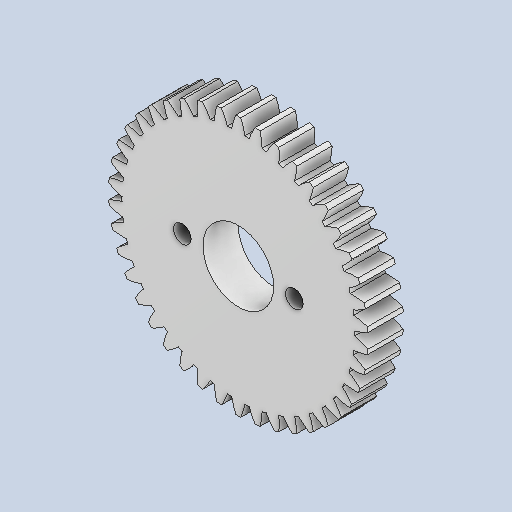
# Autodesk Inventor part: 平歯車2
Saved by Autodesk Inventor 2025.2 (Build 292293000, 293)
## iProperties
CustomPartVersion: 1
Created: 2025-01-07
Part Number: 平歯車2
Material: ABS プラスチック
Document SubType Name: Modeling
Designer: haruy
Categories: <?xml version="1.0" encoding="UTF-16"?> <MemberInstance><Categories><FamilyTemplate><FamilyTemplateParameter ValueType="xs:double" Id="1" ObjectReferenceKey="da_z" ObjectType="kUserParameterObject"/><FamilyTemplateParameter ValueType="xs:double" Id="2" ObjectReferenceKey="da_b" ObjectType="kUserParameterObject"/><FamilyTemplateParameter ValueType="xs:double" Id="3" ObjectReferenceKey="da_beta" ObjectType="kUserParameterObject"/><FamilyTemplateParameter ValueType="xs:double" Id="4" ObjectReferenceKey="da_da" ObjectType="kUserParameterObject"/><FamilyTemplateParameter ValueType="xs:double" Id="5" ObjectReferenceKey="da_aw" ObjectType="kUserParameterObject"/><FamilyTemplateParameter ValueType="xs:string" Id="6" ObjectReferenceKey="EAIAABAAAACIAQAAAAAAAIAAAAAAAAAA" ObjectType="83910656" SubObjectId="SurfaceGeometry"/></FamilyTemplate><ParamToTemplateMap><ParamToTemplate CategoryParameter="//CategoryParameter[@InternalName='046C89C9-8512-4d59-83FE-43B91F4F132A']" TemplateParameter="1"/><ParamToTemplate CategoryParameter="//CategoryParameter[@InternalName='2552DF32-E462-4b46-AEBF-C6C7768E72AC']" TemplateParameter="2"/><ParamToTemplate CategoryParameter="//CategoryParameter[@InternalName='C9EE641D-15FC-4fae-A226-E94C4372FDD7']" TemplateParameter="3"/><ParamToTemplate><ParamToTemplate CategoryParameter="//CategoryParameter[@InternalName='00B6519A-459B-49c7-AD84-2E56D39A5744']" ConstantValue="0.000000"/></ParamToTemplate><ParamToTemplate><ParamToTemplate CategoryParameter="//CategoryParameter[@InternalName='04B31F0E-C7A6-4894-AA32-9629BEFACF47']" ConstantValue="1.000000"/></ParamToTemplate><ParamToTemplate><ParamToTemplate CategoryParameter="//CategoryParameter[@InternalName='43CBEC2E-7847-49e7-A936-2F7889FCB2D9']" ConstantValue="0.250000"/></ParamToTemplate><ParamToTemplate><ParamToTemplate CategoryParameter="//CategoryParameter[@InternalName='B1EFC894-105D-4ebd-86BF-FA20ED196853']" ConstantValue="0.350000"/></ParamToTemplate><ParamToTemplate><ParamToTemplate CategoryParameter="//CategoryParameter[@InternalName='51175063-3D10-4879-93E8-6246FE8B403D']" ConstantValue="2060000000.000000"/></ParamToTemplate><ParamToTemplate><ParamToTemplate CategoryParameter="//CategoryParameter[@InternalName='A3A52E27-4454-46a9-B0BD-C932399B70AF']" ConstantValue="0.300000"/></ParamToTemplate><ParamToTemplate><ParamToTemplate CategoryParameter="//CategoryParameter[@InternalName='91B76062-C214-41d9-B1B9-14D2AB99603D']" ConstantValue="0.100000"/></ParamToTemplate><ParamToTemplate><ParamToTemplate CategoryParameter="//CategoryParameter[@InternalName='374E806E-8B8A-4dda-A9AA-1039D6500AD2']" ConstantValue="10.000000"/></ParamToTemplate><ParamToTemplate><ParamToTemplate CategoryParameter="//CategoryParameter[@InternalName='2D373A89-B862-43d6-8D0B-0CBF12AB9F6C']" ConstantValue="0.349066"/></ParamToTemplate><ParamToTemplate CategoryParameter="//CategoryParameter[@InternalName='37777632-D6A2-4fac-9D53-DB8ACD95C989']" TemplateParameter="4"/><ParamToTemplate CategoryParameter="//CategoryParameter[@InternalName='FD1017F1-B727-4f7e-9707-0F86F1FF9423']" TemplateParameter="5"/><ParamToTemplate><ParamToTemplate CategoryParameter="//CategoryParameter[@InternalName='9E1B4470-B2D3-4ff1-B813-535BB4CDF51A']" ConstantValue="3520000.000000"/></ParamToTemplate><ParamToTemplate><ParamToTemplate CategoryParameter="//CategoryParameter[@InternalName='F8452263-BFF6-458c-9FB1-07C4B99E95CD']" ConstantValue="11400000.000000"/></ParamToTemplate><ParamToTemplate><ParamToTemplate CategoryParameter="//CategoryParameter[@InternalName='3E3BB259-FD49-497f-8171-6EBC954A3479']" ConstantValue="2.000000"/></ParamToTemplate><ParamToTemplate CategoryParameter="//CategoryParameter[@InternalName='27C3BAF2-7550-4e4b-AE2C-0DB134B7D9B7']" TemplateParameter="6"/></ParamToTemplateMap><Category DisplayName="Gear" InternalName="DC85795E-93AB-48d5-8EEE-5A27447B64BD" Mnemonic="Gear"><CategoryParameter DisplayName="z" InternalName="046C89C9-8512-4d59-83FE-43B91F4F132A" Mnemonic="z"/><CategoryParameter DisplayName="b" InternalName="2552DF32-E462-4b46-AEBF-C6C7768E72AC" Mnemonic="b"/><CategoryParameter DisplayName="||b|" InternalName="C9EE641D-15FC-4fae-A226-E94C4372FDD7" Mnemonic="beta"/><CategoryParameter DisplayName="x" InternalName="00B6519A-459B-49c7-AD84-2E56D39A5744" Mnemonic="x"/><CategoryParameter DisplayName="a*" InternalName="04B31F0E-C7A6-4894-AA32-9629BEFACF47" Mnemonic="a"/><CategoryParameter DisplayName="c*" InternalName="43CBEC2E-7847-49e7-A936-2F7889FCB2D9" Mnemonic="c"/><CategoryParameter DisplayName="r|.f|*" InternalName="B1EFC894-105D-4ebd-86BF-FA20ED196853" Mnemonic="rf"/><CategoryParameter DisplayName="E" InternalName="51175063-3D10-4879-93E8-6246FE8B403D" Mnemonic="E"/><CategoryParameter DisplayName="||m|" InternalName="A3A52E27-4454-46a9-B0BD-C932399B70AF" Mnemonic="mi"/><Category DisplayName="SpurGear" InternalName="26C5A22E-A91E-4dfd-A3B3-23CCAFAE1764" Mnemonic="SpurGear"><CategoryParameter DisplayName="m" InternalName="91B76062-C214-41d9-B1B9-14D2AB99603D" Mnemonic="m"/><CategoryParameter DisplayName="P" InternalName="374E806E-8B8A-4dda-A9AA-1039D6500AD2" Mnemonic="PP"/><CategoryParameter DisplayName="||a|" InternalName="2D373A89-B862-43d6-8D0B-0CBF12AB9F6C" Mnemonic="alpha"/><CategoryParameter DisplayName="d|.a|" InternalName="37777632-D6A2-4fac-9D53-DB8ACD95C989" Mnemonic="da"/><CategoryParameter DisplayName="a|.w|" InternalName="FD1017F1-B727-4f7e-9707-0F86F1FF9423" Mnemonic="aw"/><CategoryParameter DisplayName="||s||.Flim|" InternalName="9E1B4470-B2D3-4ff1-B813-535BB4CDF51A" Mnemonic="sFlim"/><CategoryParameter DisplayName="||s||.Hlim|" InternalName="F8452263-BFF6-458c-9FB1-07C4B99E95CD" Mnemonic="sHlim"/><CategoryParameter DisplayName="タイプ" InternalName="3E3BB259-FD49-497f-8171-6EBC954A3479" Mnemonic="type"/><CategoryParameter DisplayName="PitchDiameter" InternalName="27C3BAF2-7550-4e4b-AE2C-0DB134B7D9B7" Mnemonic="IDS_PITCHDIAM"/></Category></Category></Categories></MemberInstance>
Density: 1.06 g/cm^3
Appearance: 滑らか - 白
Mass: 64.8659 g
Surface Area: 43.5022 cm^2
Volume: 8.26317 cm^3
Author: haruy
Autodesk Inventor part; units mm, degrees
ref_plane "YZ Plane" through (0, 0, 0) normal (1, 0, 0) x (0, 1, 0)
ref_plane "XZ Plane" through (0, 0, 0) normal (0, 1, 0) x (-1, 0, 0)
ref_plane "XY Plane" through (0, 0, 0) normal (0, 0, 1) x (1, 0, 0)
sketch "Sketch1" plane through (0, 0, 0) normal (0, 0, 1) x (1, 0, 0)
  circle A0 centre (0, 0) radius 22
  dimension "d0" = 44
  constraints: 1 centre point
  measures "d0" diameter of A0
extrude "Extrusion1" add sketch "Sketch1" along normal blind 6
ref_plane "Work Plane2" through (0, 0, 3) normal (0, 0, 1) x (1, 0, 0)
sketch "Sketch2" plane through (0, 0, 0) normal (0, 0, -1) x (-1, 0, 0)
  circle A0 centre (0, 0) radius 22 projected
  circle A1 centre (0, 0) radius 21
  dimension "d3" = 42
  constraints: 1 centre point, 1 coincident
  measures "d3" diameter of A1
surface extrude "ピッチ円直径" sketch "Sketch2" against normal through all shown no curves A1
ref_plane "Work Plane8" through (0, 0, 0) normal (0.9972038, 0.0747301, 0) x (0, 0, 1)
ref_plane "Work Plane9" through (0, 0, 0) normal (1, 0, 0) x (0, 1, 0)
spur gear teeth "平歯車" teeth 42 pitch diameter 42 tip diameter 44 root diameter 39.5 face width 6 start plane through (0, 0, 0) normal (0, 0, -1) x (-1, 0, 0)
sketch "スケッチ3" plane through (0, 0, 6) normal (0, 0, 1) x (1, 0, 0)
  circle A0 centre (0, 0) radius 6
  circle A1 centre (0, 0) radius 9.5
  circle A2 centre (-9.5, 0) radius 1.5
  circle A3 centre (9.5, 0) radius 1.5
  dimension "d50" = 19
  dimension "d49" = 12
  dimension "d51" = 3
  dimension "d54" = 360
  constraints: 3 centre point, 2 coincident, 1 horizontal alignment, 7 other
  measures "d49" diameter of A0
  measures "d51" diameter of A2
extrude "押し出し2" cut sketch "スケッチ3" against normal blind 10 contours A0 | A1 A3 | A1 A3 | A2 A1 | A1 A2
sketch "スケッチ4" plane through (0, 0, 6) normal (0, 0, 1) x (1, 0, 0)
  circle A0 centre (-9.5, 0) radius 1.5 projected
  circle A1 centre (9.5, 0) radius 1.5 projected
  circle A2 centre (0, 0) radius 6 projected
  arc A3 (-3.6851, 21.6892) -> (-4.034, 19.3336) centre (7.3042, 18.8581) ccw projected
  arc A4 (-4.034, 19.3336) -> (-4.7541, 19.1693) centre (0, 0) ccw projected
  arc A5 (-4.7541, 19.1693) -> (-6.0904, 21.1402) centre (-14.763, 13.8214) ccw projected
  arc A6 (-6.0904, 21.1402) -> (-6.8766, 20.8977) centre (0, 0) ccw projected
  arc A7 (-6.8766, 20.8977) -> (-6.8704, 18.5165) centre (4.4119, 19.7361) ccw projected
  arc A8 (-6.8704, 18.5165) -> (-7.558, 18.2466) centre (0, 0) ccw projected
  arc A9 (-7.558, 18.2466) -> (-9.1731, 19.9963) centre (-16.6581, 11.4667) ccw projected
  arc A10 (-9.1731, 19.9963) -> (-9.9144, 19.6394) centre (0, 0) ccw projected
  arc A11 (-9.9144, 19.6394) -> (-9.5534, 17.2857) centre (1.4211, 20.1732) ccw projected
  arc A12 (-9.5534, 17.2857) -> (-10.1931, 16.9164) centre (0, 0) ccw projected
  arc A13 (-10.1931, 16.9164) -> (-12.051, 18.4058) centre (-18.1811, 8.8559) ccw projected
  arc A14 (-12.051, 18.4058) -> (-12.7308, 17.9423) centre (0, 0) ccw projected
  arc A15 (-12.7308, 17.9423) -> (-12.023, 15.6687) centre (-1.6014, 20.1597) ccw projected
  arc A16 (-12.023, 15.6687) -> (-12.6005, 15.2082) centre (0, 0) ccw projected
  arc A17 (-12.6005, 15.2082) -> (-14.6596, 16.4041) centre (-19.2979, 6.0472) ccw projected
  arc A18 (-14.6596, 16.4041) -> (-15.2627, 15.8445) centre (0, 0) ccw projected
  arc A19 (-15.2627, 15.8445) -> (-14.2241, 13.7018) centre (-4.5882, 19.6959) ccw projected
  arc A20 (-14.2241, 13.7018) -> (-14.7264, 13.1603) centre (0, 0) ccw projected
  arc A21 (-14.7264, 13.1603) -> (-16.9408, 14.036) centre (-19.9837, 3.1035) ccw projected
  arc A22 (-16.9408, 14.036) -> (-17.4538, 13.3928) centre (0, 0) ccw projected
  arc A23 (-17.4538, 13.3928) -> (-16.1073, 11.4288) centre (-7.4725, 18.7921) ccw projected
  arc A24 (-16.1073, 11.4288) -> (-16.5234, 10.8185) centre (0, 0) ccw projected
  arc A25 (-16.5234, 10.8185) -> (-18.8435, 11.3543) centre (-20.223, 0.0904) ccw projected
  arc A26 (-18.8435, 11.3543) -> (-19.2549, 10.6418) centre (0, 0) ccw projected
  arc A27 (-19.2549, 10.6418) -> (-17.6308, 8.9004) centre (-10.1898, 17.4685) ccw projected
  arc A28 (-17.6308, 8.9004) -> (-17.9513, 8.235) centre (0, 0) ccw projected
  arc A29 (-17.9513, 8.235) -> (-20.3253, 8.419) centre (-20.0106, -2.9247) ccw projected
  arc A30 (-20.3253, 8.419) -> (-20.6259, 7.6532) centre (0, 0) ccw projected
  arc A31 (-20.6259, 7.6532) -> (-18.7604, 6.1733) centre (-12.6795, 15.7546) ccw projected
  arc A32 (-18.7604, 6.1733) -> (-18.9781, 5.4675) centre (0, 0) ccw projected
  arc A33 (-18.9781, 5.4675) -> (-21.3531, 5.2957) centre (-19.3512, -5.8745) ccw projected
  arc A34 (-21.3531, 5.2957) -> (-21.5362, 4.4935) centre (0, 0) ccw projected
  arc A35 (-21.5362, 4.4935) -> (-19.471, 3.3082) centre (-14.886, 13.6889) ccw projected
  arc A36 (-19.471, 3.3082) -> (-19.581, 2.5779) centre (0, 0) ccw projected
  arc A37 (-19.581, 2.5779) -> (-21.9039, 2.054) centre (-18.2595, -8.693) ccw projected
  arc A38 (-21.9039, 2.054) -> (-21.9654, 1.2335) centre (0, 0) ccw projected
  arc A39 (-21.9654, 1.2335) -> (-19.7465, 0.3693) centre (-16.76, 11.3174) ccw projected
  arc A40 (-19.7465, 0.3693) -> (-19.7465, -0.3693) centre (0, 0) ccw projected
  arc A41 (-19.7465, -0.3693) -> (-21.9654, -1.2335) centre (-16.76, -11.3174) ccw projected
  arc A42 (-21.9654, -1.2335) -> (-21.9039, -2.054) centre (0, 0) ccw projected
  arc A43 (-21.9039, -2.054) -> (-19.581, -2.5779) centre (-18.2595, 8.693) ccw projected
  arc A44 (-19.581, -2.5779) -> (-19.471, -3.3082) centre (0, 0) ccw projected
  arc A45 (-19.471, -3.3082) -> (-21.5362, -4.4935) centre (-14.886, -13.6889) ccw projected
  arc A46 (-21.5362, -4.4935) -> (-21.3531, -5.2957) centre (0, 0) ccw projected
  arc A47 (-21.3531, -5.2957) -> (-18.9781, -5.4675) centre (-19.3512, 5.8745) ccw projected
  arc A48 (-18.9781, -5.4675) -> (-18.7604, -6.1733) centre (0, 0) ccw projected
  arc A49 (-18.7604, -6.1733) -> (-20.6259, -7.6532) centre (-12.6795, -15.7546) ccw projected
  arc A50 (-20.6259, -7.6532) -> (-20.3253, -8.419) centre (0, 0) ccw projected
  arc A51 (-20.3253, -8.419) -> (-17.9513, -8.235) centre (-20.0106, 2.9247) ccw projected
  arc A52 (-17.9513, -8.235) -> (-17.6308, -8.9004) centre (0, 0) ccw projected
  arc A53 (-17.6308, -8.9004) -> (-19.2549, -10.6418) centre (-10.1898, -17.4685) ccw projected
  arc A54 (-19.2549, -10.6418) -> (-18.8435, -11.3543) centre (0, 0) ccw projected
  arc A55 (-18.8435, -11.3543) -> (-16.5234, -10.8185) centre (-20.223, -0.0904) ccw projected
  arc A56 (-16.5234, -10.8185) -> (-16.1073, -11.4288) centre (0, 0) ccw projected
  arc A57 (-16.1073, -11.4288) -> (-17.4538, -13.3928) centre (-7.4725, -18.7921) ccw projected
  arc A58 (-17.4538, -13.3928) -> (-16.9408, -14.036) centre (0, 0) ccw projected
  arc A59 (-16.9408, -14.036) -> (-14.7264, -13.1603) centre (-19.9837, -3.1035) ccw projected
  arc A60 (-14.7264, -13.1603) -> (-14.2241, -13.7018) centre (0, 0) ccw projected
  arc A61 (-14.2241, -13.7018) -> (-15.2627, -15.8445) centre (-4.5882, -19.6959) ccw projected
  arc A62 (-15.2627, -15.8445) -> (-14.6596, -16.4041) centre (0, 0) ccw projected
  arc A63 (-14.6596, -16.4041) -> (-12.6005, -15.2082) centre (-19.2979, -6.0472) ccw projected
  arc A64 (-12.6005, -15.2082) -> (-12.023, -15.6687) centre (0, 0) ccw projected
  arc A65 (-12.023, -15.6687) -> (-12.7308, -17.9423) centre (-1.6014, -20.1597) ccw projected
  arc A66 (-12.7308, -17.9423) -> (-12.051, -18.4058) centre (0, 0) ccw projected
  arc A67 (-12.051, -18.4058) -> (-10.1931, -16.9164) centre (-18.1811, -8.8559) ccw projected
  arc A68 (-10.1931, -16.9164) -> (-9.5534, -17.2857) centre (0, 0) ccw projected
  arc A69 (-9.5534, -17.2857) -> (-9.9144, -19.6394) centre (1.4211, -20.1732) ccw projected
  arc A70 (-9.9144, -19.6394) -> (-9.1731, -19.9963) centre (0, 0) ccw projected
  arc A71 (-9.1731, -19.9963) -> (-7.558, -18.2466) centre (-16.6581, -11.4667) ccw projected
  arc A72 (-7.558, -18.2466) -> (-6.8704, -18.5165) centre (0, 0) ccw projected
  arc A73 (-6.8704, -18.5165) -> (-6.8766, -20.8977) centre (4.4119, -19.7361) ccw projected
  arc A74 (-6.8766, -20.8977) -> (-6.0904, -21.1402) centre (0, 0) ccw projected
  arc A75 (-6.0904, -21.1402) -> (-4.7541, -19.1693) centre (-14.763, -13.8214) ccw projected
  arc A76 (-4.7541, -19.1693) -> (-4.034, -19.3336) centre (0, 0) ccw projected
  arc A77 (-4.034, -19.3336) -> (-3.6851, -21.6892) centre (7.3042, -18.8581) ccw projected
  arc A78 (-3.6851, -21.6892) -> (-2.8716, -21.8118) centre (0, 0) ccw projected
  arc A79 (-2.8716, -21.8118) -> (-1.8439, -19.6637) centre (-12.5382, -15.8674) ccw projected
  arc A80 (-1.8439, -19.6637) -> (-1.1074, -19.7189) centre (0, 0) ccw projected
  arc A81 (-1.1074, -19.7189) -> (-0.4114, -21.9962) centre (10.0332, -17.5589) ccw projected
  arc A82 (-0.4114, -21.9962) -> (0.4114, -21.9962) centre (0, 0) ccw projected
  arc A83 (0.4114, -21.9962) -> (1.1074, -19.7189) centre (-10.0332, -17.5589) ccw projected
  arc A84 (1.1074, -19.7189) -> (1.8439, -19.6637) centre (0, 0) ccw projected
  arc A85 (1.8439, -19.6637) -> (2.8716, -21.8118) centre (12.5382, -15.8674) ccw projected
  arc A86 (2.8716, -21.8118) -> (3.6851, -21.6892) centre (0, 0) ccw projected
  arc A87 (3.6851, -21.6892) -> (4.034, -19.3336) centre (-7.3042, -18.8581) ccw projected
  arc A88 (4.034, -19.3336) -> (4.7541, -19.1693) centre (0, 0) ccw projected
  arc A89 (4.7541, -19.1693) -> (6.0904, -21.1402) centre (14.763, -13.8214) ccw projected
  arc A90 (6.0904, -21.1402) -> (6.8766, -20.8977) centre (0, 0) ccw projected
  arc A91 (6.8766, -20.8977) -> (6.8704, -18.5165) centre (-4.4119, -19.7361) ccw projected
  arc A92 (6.8704, -18.5165) -> (7.558, -18.2466) centre (0, 0) ccw projected
  arc A93 (7.558, -18.2466) -> (9.1731, -19.9963) centre (16.6581, -11.4667) ccw projected
  arc A94 (9.1731, -19.9963) -> (9.9144, -19.6394) centre (0, 0) ccw projected
  arc A95 (9.9144, -19.6394) -> (9.5534, -17.2857) centre (-1.4211, -20.1732) ccw projected
  arc A96 (9.5534, -17.2857) -> (10.1931, -16.9164) centre (0, 0) ccw projected
  arc A97 (10.1931, -16.9164) -> (12.051, -18.4058) centre (18.1811, -8.8559) ccw projected
  arc A98 (12.051, -18.4058) -> (12.7308, -17.9423) centre (0, 0) ccw projected
  arc A99 (12.7308, -17.9423) -> (12.023, -15.6687) centre (1.6014, -20.1597) ccw projected
  arc A100 (12.023, -15.6687) -> (12.6005, -15.2082) centre (0, 0) ccw projected
  arc A101 (12.6005, -15.2082) -> (14.6596, -16.4041) centre (19.2979, -6.0472) ccw projected
  arc A102 (14.6596, -16.4041) -> (15.2627, -15.8445) centre (0, 0) ccw projected
  arc A103 (15.2627, -15.8445) -> (14.2241, -13.7018) centre (4.5882, -19.6959) ccw projected
  arc A104 (14.2241, -13.7018) -> (14.7264, -13.1603) centre (0, 0) ccw projected
  arc A105 (14.7264, -13.1603) -> (16.9408, -14.036) centre (19.9837, -3.1035) ccw projected
  arc A106 (16.9408, -14.036) -> (17.4538, -13.3928) centre (0, 0) ccw projected
  arc A107 (17.4538, -13.3928) -> (16.1073, -11.4288) centre (7.4725, -18.7921) ccw projected
  arc A108 (16.1073, -11.4288) -> (16.5234, -10.8185) centre (0, 0) ccw projected
  arc A109 (16.5234, -10.8185) -> (18.8435, -11.3543) centre (20.223, -0.0904) ccw projected
  arc A110 (18.8435, -11.3543) -> (19.2549, -10.6418) centre (0, 0) ccw projected
  arc A111 (19.2549, -10.6418) -> (17.6308, -8.9004) centre (10.1898, -17.4685) ccw projected
  arc A112 (17.6308, -8.9004) -> (17.9513, -8.235) centre (0, 0) ccw projected
  arc A113 (17.9513, -8.235) -> (20.3253, -8.419) centre (20.0106, 2.9247) ccw projected
  arc A114 (20.3253, -8.419) -> (20.6259, -7.6532) centre (0, 0) ccw projected
  arc A115 (20.6259, -7.6532) -> (18.7604, -6.1733) centre (12.6795, -15.7546) ccw projected
  arc A116 (18.7604, -6.1733) -> (18.9781, -5.4675) centre (0, 0) ccw projected
  arc A117 (18.9781, -5.4675) -> (21.3531, -5.2957) centre (19.3512, 5.8745) ccw projected
  arc A118 (21.3531, -5.2957) -> (21.5362, -4.4935) centre (0, 0) ccw projected
  arc A119 (21.5362, -4.4935) -> (19.471, -3.3082) centre (14.886, -13.6889) ccw projected
  arc A120 (19.471, -3.3082) -> (19.581, -2.5779) centre (0, 0) ccw projected
  arc A121 (19.581, -2.5779) -> (21.9039, -2.054) centre (18.2595, 8.693) ccw projected
  arc A122 (21.9039, -2.054) -> (21.9654, -1.2335) centre (0, 0) ccw projected
  arc A123 (21.9654, -1.2335) -> (19.7465, -0.3693) centre (16.76, -11.3174) ccw projected
  arc A124 (19.7465, -0.3693) -> (19.7465, 0.3693) centre (0, 0) ccw projected
  arc A125 (19.7465, 0.3693) -> (21.9654, 1.2335) centre (16.76, 11.3174) ccw projected
  arc A126 (21.9654, 1.2335) -> (21.9039, 2.054) centre (0, 0) ccw projected
  arc A127 (21.9039, 2.054) -> (19.581, 2.5779) centre (18.2595, -8.693) ccw projected
  arc A128 (19.581, 2.5779) -> (19.471, 3.3082) centre (0, 0) ccw projected
  arc A129 (19.471, 3.3082) -> (21.5362, 4.4935) centre (14.886, 13.6889) ccw projected
  arc A130 (21.5362, 4.4935) -> (21.3531, 5.2957) centre (0, 0) ccw projected
  arc A131 (21.3531, 5.2957) -> (18.9781, 5.4675) centre (19.3512, -5.8745) ccw projected
  arc A132 (18.9781, 5.4675) -> (18.7604, 6.1733) centre (0, 0) ccw projected
  arc A133 (18.7604, 6.1733) -> (20.6259, 7.6532) centre (12.6795, 15.7546) ccw projected
  arc A134 (20.6259, 7.6532) -> (20.3253, 8.419) centre (0, 0) ccw projected
  arc A135 (20.3253, 8.419) -> (17.9513, 8.235) centre (20.0106, -2.9247) ccw projected
  arc A136 (17.9513, 8.235) -> (17.6308, 8.9004) centre (0, 0) ccw projected
  arc A137 (17.6308, 8.9004) -> (19.2549, 10.6418) centre (10.1898, 17.4685) ccw projected
  arc A138 (19.2549, 10.6418) -> (18.8435, 11.3543) centre (0, 0) ccw projected
  arc A139 (18.8435, 11.3543) -> (16.5234, 10.8185) centre (20.223, 0.0904) ccw projected
  arc A140 (16.5234, 10.8185) -> (16.1073, 11.4288) centre (0, 0) ccw projected
  arc A141 (16.1073, 11.4288) -> (17.4538, 13.3928) centre (7.4725, 18.7921) ccw projected
  arc A142 (17.4538, 13.3928) -> (16.9408, 14.036) centre (0, 0) ccw projected
  arc A143 (16.9408, 14.036) -> (14.7264, 13.1603) centre (19.9837, 3.1035) ccw projected
  arc A144 (14.7264, 13.1603) -> (14.2241, 13.7018) centre (0, 0) ccw projected
  arc A145 (14.2241, 13.7018) -> (15.2627, 15.8445) centre (4.5882, 19.6959) ccw projected
  arc A146 (15.2627, 15.8445) -> (14.6596, 16.4041) centre (0, 0) ccw projected
  arc A147 (14.6596, 16.4041) -> (12.6005, 15.2082) centre (19.2979, 6.0472) ccw projected
  arc A148 (12.6005, 15.2082) -> (12.023, 15.6687) centre (0, 0) ccw projected
  arc A149 (12.023, 15.6687) -> (12.7308, 17.9423) centre (1.6014, 20.1597) ccw projected
  arc A150 (12.7308, 17.9423) -> (12.051, 18.4058) centre (0, 0) ccw projected
  arc A151 (12.051, 18.4058) -> (10.1931, 16.9164) centre (18.1811, 8.8559) ccw projected
  arc A152 (10.1931, 16.9164) -> (9.5534, 17.2857) centre (0, 0) ccw projected
  arc A153 (9.5534, 17.2857) -> (9.9144, 19.6394) centre (-1.4211, 20.1732) ccw projected
  arc A154 (9.9144, 19.6394) -> (9.1731, 19.9963) centre (0, 0) ccw projected
  arc A155 (9.1731, 19.9963) -> (7.558, 18.2466) centre (16.6581, 11.4667) ccw projected
  arc A156 (7.558, 18.2466) -> (6.8704, 18.5165) centre (0, 0) ccw projected
  arc A157 (6.8704, 18.5165) -> (6.8766, 20.8977) centre (-4.4119, 19.7361) ccw projected
  arc A158 (6.8766, 20.8977) -> (6.0904, 21.1402) centre (0, 0) ccw projected
  arc A159 (6.0904, 21.1402) -> (4.7541, 19.1693) centre (14.763, 13.8214) ccw projected
  arc A160 (4.7541, 19.1693) -> (4.034, 19.3336) centre (0, 0) ccw projected
  arc A161 (4.034, 19.3336) -> (3.6851, 21.6892) centre (-7.3042, 18.8581) ccw projected
  arc A162 (3.6851, 21.6892) -> (2.8716, 21.8118) centre (0, 0) ccw projected
  arc A163 (2.8716, 21.8118) -> (1.8439, 19.6637) centre (12.5382, 15.8674) ccw projected
  arc A164 (1.8439, 19.6637) -> (1.1074, 19.7189) centre (0, 0) ccw projected
  arc A165 (1.1074, 19.7189) -> (0.4114, 21.9962) centre (-10.0332, 17.5589) ccw projected
  arc A166 (0.4114, 21.9962) -> (-0.4114, 21.9962) centre (0, 0) ccw projected
  arc A167 (-0.4114, 21.9962) -> (-1.1074, 19.7189) centre (10.0332, 17.5589) ccw projected
  arc A168 (-1.1074, 19.7189) -> (-1.8439, 19.6637) centre (0, 0) ccw projected
  arc A169 (-1.8439, 19.6637) -> (-2.8716, 21.8118) centre (-12.5382, 15.8674) ccw projected
  arc A170 (-2.8716, 21.8118) -> (-3.6851, 21.6892) centre (0, 0) ccw projected
equation "\"d0\" = da_da"
equation "\"d1\" = da_b"
equation "\"d3\" = da_d"
equation "\"d16\" = da_aw"
equation "\"d43\" = da_aw"
equation "\"d46\" = da_aw"
equation "\"da_da\" = 44"
equation "\"da_b\" = 6"
equation "\"da_d\" = 42"
equation "\"da_aw\" = 42"
body "Solid1"
body "Srf1"
